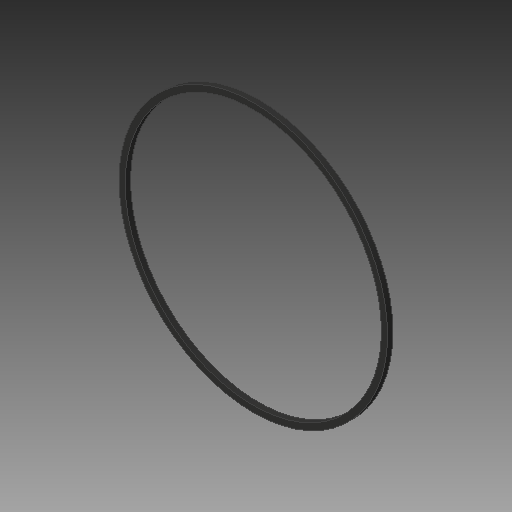
# Autodesk Inventor part: 1135_Sq O Ring_V1
Saved by Autodesk Inventor 2020 (Build 240168000, 168)
## iProperties
Created: 2019-05-13
Part Number: 1135_Sq O Ring_V1
Material: Rubber
Document SubType Name: Modeling
Designer: e22ma
Density: 0.93 g/cm^3
Appearance: Rubber - Black
Author: e22ma
Autodesk Inventor part; units mm, degrees
ref_plane "YZ Plane" through (0, 0, 0) normal (1, 0, 0) x (0, 1, 0)
ref_plane "XZ Plane" through (0, 0, 0) normal (0, 1, 0) x (-1, 0, 0)
ref_plane "Work Plane1" through (0, 0, 0) normal (0, 0, 1) x (1, 0, 0)
sketch "Sketch1" plane through (0, 0, 0) normal (0, 0, 1) x (1, 0, 0)
  circle A0 centre (80.1116, 0) radius 76.454 projected
  circle A1 centre (80.1116, 0) radius 80.1116 projected
  point P0 (0, 0)
  constraints: 1 horizontal alignment
extrude "Extrusion1" add sketch "Sketch1" along normal blind 3.175
body "Solid1"
